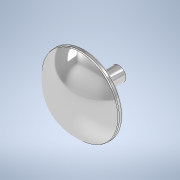
# Autodesk Inventor part: Round Knob
Saved by Autodesk Inventor 2022 (Build 260153000, 153)
## iProperties
Company: Jay's Dressers
Created: 2021-10-04
Material: Generic
Document SubType Name: Modeling
Designer: Admin
Density: 1 g/cm^3
Appearance: Chrome - Polished
Author: Admin
Title: Round Knob
Autodesk Inventor part; units mm, degrees
ref_plane "YZ Plane" through (0, 0, 0) normal (1, 0, 0) x (0, 1, 0)
ref_plane "XZ Plane" through (0, 0, 0) normal (0, 1, 0) x (-1, 0, 0)
ref_plane "XY Plane" through (0, 0, 0) normal (0, 0, 1) x (1, 0, 0)
sketch "Sketch1" plane through (0, 0, 0) normal (1, 0, 0) x (0, 1, 0)
  line L0 (0, 0) -> (0, 38.1)
  arc A0 (25.4, 25.4) -> (0, 38.1) centre (0, 6.35) ccw
  line L1 (25.4, 25.4) -> (25.4, 22.225)
  line L2 (25.4, 22.225) -> (4.7625, 22.225)
  line L3 (4.7625, 22.225) -> (4.7625, 0)
  line L4 (4.7625, 0) -> (0, 0)
  dimension "d0" = 9.525
  dimension "d1" = 38.1
  dimension "d2" = 22.225
  dimension "d3" = 50.8
  dimension "d4" = 3.175
  constraints: 10 end point, 3 perpendicular, 2 point on circle, 1 centre point, 1 parallel, 1 point on line, 1 vertical
  measures "d0" diameter of L3 L0
  measures "d1" distance of L0.start L0.end
  measures "d2" distance of L2.end L3.end
  measures "d3" diameter of L1 L0
  measures "d4" distance of L1.start L1.end
revolve "Revolution1" add sketch "Sketch1" angle 360 about axis through (0, 0, 0) along (0, 0, 1)
fillet "Fillet1" radius 1.27 2 edges at (0, -25.4, 22.225) (0, -25.4, 25.4)
body "Solid1"
